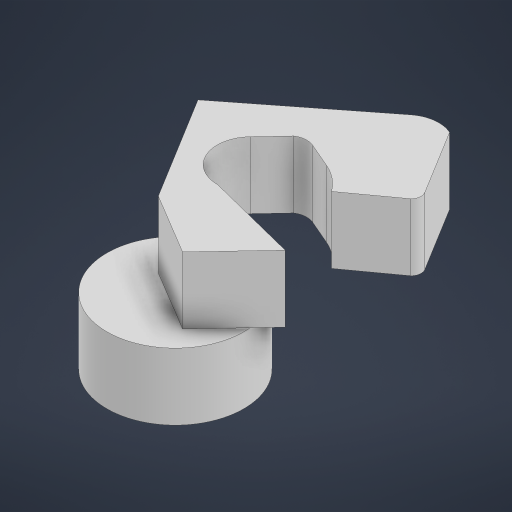
# Autodesk Inventor part: Test part
Saved by Autodesk Inventor 2024.1 (Build 281209000, 209)
## iProperties
Created: 2024-01-22
Part Number: Test part
Material: Generic
Document SubType Name: Modeling
Designer: vg3
Density: 1 g/cm^3
Appearance: Default
Author: vg3
Autodesk Inventor part; units mm, degrees
ref_plane "YZ Plane" through (0, 0, 0) normal (1, 0, 0) x (0, 1, 0)
ref_plane "XZ Plane" through (0, 0, 0) normal (0, 1, 0) x (-1, 0, 0)
ref_plane "XY Plane" through (0, 0, 0) normal (0, 0, 1) x (1, 0, 0)
sketch "Sketch1" plane through (0, 0, 0) normal (0, 1, 0) x (-1, 0, 0)
  circle A0 centre (4.6155, 11.5612) radius 26.0349
  point P0 (0, 0)
  constraints: 1 centre point
extrude "Extrusion1" add sketch "Sketch1" along normal blind 25.4
sketch "Sketch2" plane through (-4.6155, 25.4, 11.5612) normal (0, 1, 0) x (1, 0, 0)
  line L0 (-9.602, 3.1232) -> (-33.7988, 42.4236)
  line L1 (-33.7988, 42.4236) -> (11.6664, 78.0251)
  arc A0 (24.8436, 79.6434) -> (11.6664, 78.0251) centre (19.5984, 67.8956) ccw
  line L2 (24.8436, 79.6434) -> (39.9619, 55.0882)
  arc A1 (39.4079, 50.3607) -> (39.9619, 55.0882) centre (36.6923, 53.0751) ccw
  line L3 (39.4079, 50.3607) -> (21.8383, 37.6459)
  arc A2 (21.8383, 37.6459) -> (12.1988, 45.3621) centre (3.0409, 24.0425) ccw
  line L4 (12.1988, 45.3621) -> (3.0438, 49.2947)
  arc A3 (3.0438, 49.2947) -> (-3.6684, 48.7425) centre (0.208, 42.6931) ccw
  line L5 (-3.6684, 48.7425) -> (-11.7064, 40.2083)
  arc A4 (-11.7064, 40.2083) -> (-2.2121, 18.2269) centre (-2.2136, 31.2674) ccw
  line L6 (-2.2121, 18.2269) -> (32.4028, 9.4421)
  line L7 (32.4028, 9.4421) -> (13.4408, -10.6903)
  line L8 (13.4408, -10.6903) -> (-9.602, 3.1232)
  point P0 (4.6155, 11.5612)
  constraints: 18 end point, 10 point on circle, 5 centre point, 5 tangent, 2 parallel, 1 point on line
extrude "Extrusion2" add sketch "Sketch2" along normal blind 25.4
body "Solid1"
